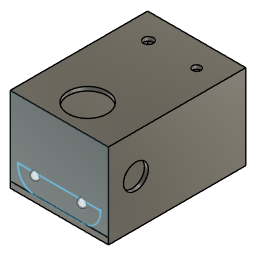
Fuzz Buddy3dModel (Autodesk Fusion 360 design; units mm, degrees)
Autodesk Fusion 360 part; units mm, degrees
note: some values were not read from the file. Chosen so that the rebuilt part matches the saved one: which bodies a step acts on; which face or edge a step refers to.
box "BoxPrimitive1" add length 35 width 25 height 20 placed x (0, 1, 0) y (-1, 0, 0) z (0, 0, 1) at (25, 0, 0) makes body 1
shell "Shell1" thickness 1 removed faces 1 at (8.3333, 11.6667, 0) on bodies 1
hole "Hole1" at (25, 7.0112, 10.0205) direction (-1, 0, 0) diameter 6.35 depth 25 tip angle 180 bodies 1
hole "Hole2" at (13.1055, 35, 10.2564) direction (0, -1, 0) diameter 2.1 depth 15 tip angle 180 bodies 1
hole "Hole3" at (12.5231, 7.194, 20) direction (0, 0, -1) diameter 10 depth 10 tip angle 180 bodies 1
hole "Hole4" at (18.8192, 28.6638, 20) direction (0, 0, -1) diameter 2.1 depth 10 tip angle 180 bodies 1
hole "Hole5" at (6.6036, 28.6103, 20) direction (0, 0, -1) diameter 2.5 depth 10 tip angle 180 bodies 1
sketch "Sketch3" plane through (0, 0, 0) normal (0, -1, 0) x (1, 0, 0)
  line L0 (0, 20) -> (0, 0)
  line L1 (0, 0) -> (25, 0)
  line L2 (25, 0) -> (25, 20)
  line L3 (25, 20) -> (0, 20)
  line L4 (2, 5) -> (23, 5)
  line L5 (23, 5) -> (23, 4.5)
  line L6 (18.5, 0) -> (6.5, 0)
  line L7 (2, 4.5) -> (2, 5)
  arc A0 (2, 4.5) -> (6.5, 0) centre (6.5, 4.5) ccw
  arc A1 (18.5, 0) -> (23, 4.5) centre (18.5, 4.5) ccw
  dimension "d22" = 4.5
  constraint horizontal L4
  constraint vertical L5
  constraint horizontal L6
  constraint vertical L7
  constraint tangent L6 A0
  constraint tangent L7 A0
  constraint tangent L5 A1
  constraint tangent L6 A1
  constraint equal A0 A1
  measures "d22" radius of A0
sketch "Sketch4" plane through (0, 0, 0) normal (0, 0, 1) x (1, 0, 0)
sketch "Sketch5" plane through (0, 0, 0) normal (1, 0, 0) x (0, 1, 0)
  line L0 (30.6743, -10.5966) -> (4.8, -10.5966)
  line L1 (4.8, -10.5966) -> (4.8, -9.55)
  line L2 (4.8, -9.55) -> (30.6743, -9.55)
  line L3 (30.6743, -9.55) -> (30.6743, -10.5966)
  constraint horizontal L0
  constraint vertical L1
  constraint horizontal L2
  constraint vertical L3
extrude "Extrude1" add sketch "Sketch5" along normal blind 12 separate body makes body 2
extrude "Extrude2" add 1 faces at (4, 4.8, -10.2477) along direction (0, -1, 0) blind 4.8 on bodies 2 bodies 2
extrude "Extrude3" add 1 faces at (4, 30.6743, -9.8989) along direction (0, 1, 0) blind 4.3 on bodies 2 bodies 2
extrude "Extrude4" add 1 faces at (12, 23.3162, -10.2477) along direction (1, 0, 0) blind 13 on bodies 2 bodies 2
move_face "MoveFace1" by (0, 0, 1) 1 faces at (16.6667, 23.3162, -9.55) on bodies 2
move_body "Move1" bodies 2 to x (1, 0, 0) y (0, 1, 0) z (0, 0, 1) at (0, 0, 8.5)
combine "Combine1" operation add target body 1 tool bodies 2 makes body 3 at (8.3333, 11.6581, -0.05)
move_body "Align1" bodies 3 to x (1, 0, 0) y (0, 1, 0) z (0, 0, 1) at (0, 0.0257, 0)
combine "Combine2" operation add target body 3 tool bodies 1 makes body 4 at (12.7349, 22.5614, 20)
move_body "Move2" bodies 3 to x (1, 0, 0) y (0, 1, 0) z (0, 0, 1) at (0, 0, 0.5)
combine "Combine3" operation add target body 3 tool bodies 4
